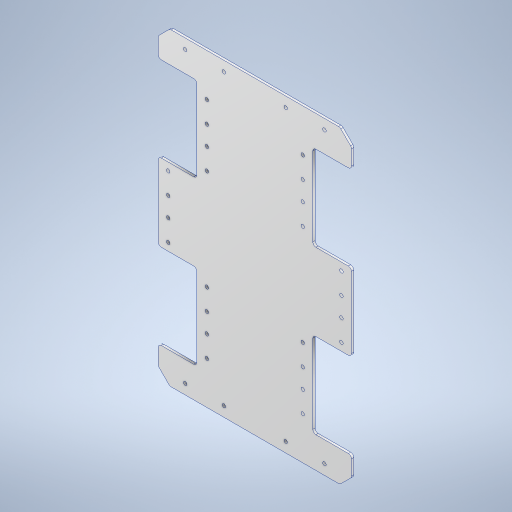
# Autodesk Inventor part: Grundgehäuse_01
Saved by Autodesk Inventor 2024 (Build 280153000, 153)
## iProperties
Created: 2024-03-13
Part Number: Grundgehäuse_01
Material: Aluminium 6061
Document SubType Name: Modellieren
Designer: month
Density: 2.7 g/cm^3
Appearance: Aluminium - flach
Sheet Metal Rule: Standard
Author: month
Autodesk Inventor part; units mm, degrees
ref_plane "YZ Plane" through (0, 0, 0) normal (1, 0, 0) x (0, 1, 0)
ref_plane "XZ Plane" through (0, 0, 0) normal (0, 1, 0) x (-1, 0, 0)
ref_plane "XY Plane" through (0, 0, 0) normal (0, 0, 1) x (1, 0, 0)
sketch "Skizze1" plane through (0, 0, 0) normal (0, 1, 0) x (-1, 0, 0)
  line L0 (0, 0) -> (250, 0)
  line L1 (250, 0) -> (250, -400)
  line L2 (250, -400) -> (0, -400)
  line L3 (0, -400) -> (0, 0)
  dimension "d0" = 400
  dimension "d1" = 250
  constraints: 8 end point, 2 parallel, 1 horizontal, 1 perpendicular
  measures "d0" distance of L2.end L0.start
  measures "d1" distance of L0.start L0.end
extrude "Extrusion1" add sketch "Skizze1" along normal blind 3
sketch "Skizze7" plane through (0, 3, 0) normal (0, 1, 0) x (1, 0, 0)
  line L0 (-250, 400) -> (-250, 0) projected
  line L1 (-250, 15) -> (-235, 0)
  line L2 (-250, 0) -> (0, 0) projected
  line L3 (-250, 15) -> (-250, 0)
  line L4 (-250, 0) -> (-235, 0)
  line L5 (0, 0) -> (0, 400) projected
  line L6 (0, 0) -> (-15, 0)
  line L7 (-15, 0) -> (0, 15)
  line L8 (-250, 400) -> (-250, 0) projected
  line L9 (-250, 200) -> (0, 200)
  line L10 (0, 0) -> (0, 400) projected
  line L11 (-125, 0) -> (-125, 400)
  line L12 (0, 400) -> (-250, 400) projected
  line L13 (0, 0) -> (0, 15)
  line L14 (-250, 385) -> (-235, 400)
  line L15 (-250, 385) -> (-250, 400)
  line L16 (-250, 400) -> (-235, 400)
  line L17 (0, 400) -> (-15, 400)
  line L18 (-15, 400) -> (0, 385)
  line L19 (0, 400) -> (0, 385)
  point P0 (-200, 30)
  point P1 (0, 30)
  point P2 (-200, 290)
  point P3 (-200, 110)
  point P4 (0, 110)
  point P5 (0, 290)
  point P6 (-235, 400)
  point P7 (-15, 400)
  point P8 (-15, 0)
  dimension "d57" = 15
  dimension "d58" = 15
  constraints: 28 end point, 6 symmetric about line, 4 point on line, 3 midpoint, 1 collinear, 1 perpendicular, 1 vertical, 4 other
  measures "d57" distance of L2.start L1.end
  measures "d58" distance of L2.start L1.start
extrude "Extrusion7" cut sketch "Skizze7" against normal blind 10 contours L12 L14 L0 | L1 L2 L0 | L12 L5 L18 | L5 L2 L7
sketch "Skizze6" plane through (0, 3, 0) normal (0, 1, 0) x (1, 0, 0)
  line L0 (-200, 40) -> (-200, 40)
  line L1 (-250, 0) -> (0, 0) projected
  line L2 (0, 400) -> (-250, 400) projected
  line L3 (0, 40) -> (0, 40)
  line L4 (-250, 400) -> (-250, 0) projected
  line L5 (-250, 250) -> (-200, 250)
  line L6 (-200, 250) -> (-200, 360)
  line L7 (-200, 360) -> (-250, 360)
  line L8 (-250, 360) -> (-250, 250)
  line L9 (-125, 400) -> (-125, 0)
  line L10 (0, 0) -> (0, 400) projected
  line L11 (0, 200) -> (-250, 200)
  line L12 (0, 400) -> (0, 0)
  line L13 (0, 250) -> (-50, 250)
  line L14 (-50, 250) -> (-50, 360)
  line L15 (-50, 360) -> (0, 360)
  line L16 (-250, 0) -> (-250, 400)
  line L17 (-250, 150) -> (-200, 150)
  line L18 (-200, 150) -> (-200, 40)
  line L19 (-200, 40) -> (-250, 40)
  line L20 (0, 400) -> (0, 0)
  line L21 (-50, 40) -> (0, 40)
  line L22 (-50, 150) -> (-50, 40)
  line L23 (0, 150) -> (-50, 150)
  point P0 (-25, 40)
  point P1 (0, 250)
  point P2 (0, 360)
  point P3 (0, 150)
  dimension "d74" = 110
  dimension "d75" = 40
  dimension "d76" = 50
  dimension "d77" = 110
  dimension "d78" = 50
  dimension "d79" = 110
  dimension "d80" = 50
  constraints: 40 end point, 14 symmetric about line, 4 midpoint, 2 parallel, 2 point on line, 1 horizontal, 1 perpendicular, 3 other
  measures "d74" distance between parallel lines of L7 L5
  measures "d75" distance between parallel lines of L2 L7
  measures "d77" distance of L18.start L0.end
  measures "d78" distance of L22.end L3.end
  measures "d79" distance from line of L23 point (-25, 40)
  measures "d80" distance of L0.end L19.end
extrude "Extrusion11" cut sketch "Skizze6" against normal blind 10 contours L4 L17 L18 L19 | L21 L22 L23 L10 | L13 L14 L15 L10 | L4 L7 L6 L5
sketch "Skizze9" plane through (0, 3, 0) normal (0, 1, 0) x (1, 0, 0)
  line L0 (-235, 0) -> (-15, 0) projected
  line L1 (-125, 0) -> (-125, 400)
  line L2 (-15, 400) -> (-235, 400) projected
  line L3 (0, 150) -> (0, 250) projected
  line L4 (0, 200) -> (-250, 200)
  line L5 (-250, 250) -> (-250, 150) projected
  line L6 (-200, 250) -> (-250, 250) projected
  line L7 (-237, 250) -> (-237, 150) construction
  circle A0 centre (-237, 240) radius 2.25
  circle A1 centre (-237, 212.5) radius 2.25
  circle A2 centre (-237, 187.5) radius 2.25
  circle A3 centre (-237, 160) radius 2.25
  circle A4 centre (-13, 240) radius 2.25
  circle A5 centre (-13, 212.5) radius 2.25
  circle A6 centre (-13, 187.5) radius 2.25
  circle A7 centre (-13, 160) radius 2.25
  line L8 (-187, 400) -> (-187, 0) construction
  line L9 (-200, 150) -> (-200, 40) projected
  circle A8 centre (-187, 55) radius 2.25
  circle A9 centre (-187, 82.5) radius 2.25
  circle A10 centre (-187, 107.5) radius 2.25
  circle A11 centre (-187, 135) radius 2.25
  line L10 (-50, 40) -> (-50, 150) projected
  line L11 (-50, 95) -> (-200, 95) construction
  circle A12 centre (-63, 55) radius 2.25
  circle A13 centre (-63, 82.5) radius 2.25
  circle A14 centre (-63, 107.5) radius 2.25
  circle A15 centre (-63, 135) radius 2.25
  circle A16 centre (-187, 345) radius 2.25
  circle A17 centre (-187, 317.5) radius 2.25
  circle A18 centre (-187, 292.5) radius 2.25
  circle A19 centre (-187, 265) radius 2.25
  circle A20 centre (-63, 345) radius 2.25
  circle A21 centre (-63, 317.5) radius 2.25
  circle A22 centre (-63, 292.5) radius 2.25
  circle A23 centre (-63, 265) radius 2.25
  line L12 (0, 15) -> (0, 40) projected
  line L13 (0, 13) -> (-250, 13) construction
  line L14 (-250, 40) -> (-250, 15) projected
  circle A24 centre (-35, 13) radius 2.25
  circle A25 centre (-85, 13) radius 2.25
  circle A26 centre (-165, 13) radius 2.25
  circle A27 centre (-215, 13) radius 2.25
  circle A28 centre (-35, 387) radius 2.25
  circle A29 centre (-85, 387) radius 2.25
  circle A30 centre (-165, 387) radius 2.25
  circle A31 centre (-215, 387) radius 2.25
  point P0 (0, 0)
  dimension "d85" = 13
  dimension "d86" = 4.5
  dimension "d87" = 4.5
  dimension "d88" = 4.5
  dimension "d89" = 4.5
  dimension "d90" = 25
  dimension "d91" = 80
  dimension "d92" = 13
  dimension "d93" = 4.5
  dimension "d94" = 4.5
  dimension "d95" = 4.5
  dimension "d96" = 4.5
  dimension "d97" = 25
  dimension "d98" = 80
  dimension "d99" = 13
  dimension "d100" = 4.5
  dimension "d101" = 4.5
  dimension "d102" = 4.5
  dimension "d103" = 4.5
  dimension "d104" = 80
  dimension "d105" = 180
  constraints: 32 centre point, 26 symmetric about line, 17 point on line, 12 end point, 6 midpoint, 1 horizontal, 1 perpendicular, 1 vertical, 20 other
  measures "d85" distance between parallel lines of L5 L7
  measures "d86" diameter of A3
  measures "d87" diameter of A2
  measures "d88" diameter of A1
  measures "d89" diameter of A0
  measures "d90" distance of A1.centre A2.centre
  measures "d91" distance of A0.centre A3.centre
  measures "d92" distance between parallel lines of L8 L9
  measures "d93" diameter of A8
  measures "d94" diameter of A9
  measures "d95" diameter of A10
  measures "d96" diameter of A11
  measures "d97" distance of A9.centre A10.centre
  measures "d98" distance of A8.centre A11.centre
  measures "d99" distance between parallel lines of L13 L0
  measures "d100" diameter of A25
  measures "d101" diameter of A24
  measures "d102" diameter of A26
  measures "d103" diameter of A27
  measures "d104" distance of A26.centre A25.centre
  measures "d105" distance of A27.centre A24.centre
extrude "Extrusion12" cut sketch "Skizze9" against normal blind 10
fillet "Rundung1" radius 4 24 edges at (-235, 1.5, -400) (-250, 1.5, -385) (-250, 1.5, -360) (-200, 1.5, -360) (-200, 1.5, -250) (-250, 1.5, -250) (-250, 1.5, -150) (-200, 1.5, -150) (-250, 1.5, -40) (-200, 1.5, -40) (-250, 1.5, -15) (-235, 1.5, 0) (-15, 1.5, 0) (0, 1.5, -15) (0, 1.5, -40) (-50, 1.5, -150) (0, 1.5, -150) (-50, 1.5, -40) (0, 1.5, -250) (-50, 1.5, -250) (-15, 1.5, -400) (0, 1.5, -385) (0, 1.5, -360) (-50, 1.5, -360)
equation "\"Biegeradius\" = Stärke"
equation "\"BreiteBiegungsfreistellung\" = Stärke"
equation "\"TiefeBiegungsfreistellung\" = 0.5 * Stärke"
equation "\"GrößeEckenfreistellung\" = 4 * Stärke"
equation "\"MinimalRest\" = 2 * Stärke"
equation "\"Übergangsradius\" = Biegeradius"
equation "\"JacobiRadiusGröße\" = Biegeradius"
equation "\"Abstandsgröße\" = Stärke"
equation "\"Stärke\" = 3.048"
